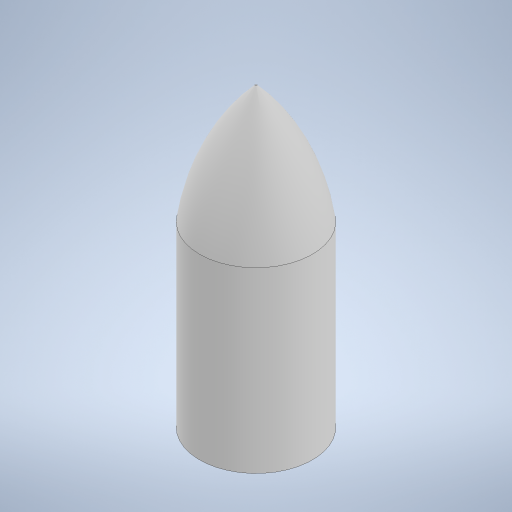
# Autodesk Inventor part: 물로켓탄두1
Saved by Autodesk Inventor 2023 (Build 270158000, 158)
## iProperties
Created: 2023-08-29
Part Number: 물로켓탄두1
Material: 일반
Document SubType Name: Modeling
Designer: rlatk
Density: 1 g/cm^3
Appearance: 기본값
Author: rlatk
Autodesk Inventor part; units mm, degrees
ref_plane "YZ Plane" through (0, 0, 0) normal (1, 0, 0) x (0, 1, 0)
ref_plane "XZ Plane" through (0, 0, 0) normal (0, 1, 0) x (-1, 0, 0)
ref_plane "XY Plane" through (0, 0, 0) normal (0, 0, 1) x (1, 0, 0)
sketch "스케치1" plane through (0, 0, 0) normal (0, 1, 0) x (-1, 0, 0)
  circle A0 centre (0, 0) radius 45.5
  circle A1 centre (0, 0) radius 47.5
  dimension "d0" = 91
  dimension "d1" = 2
  constraints: 2 centre point, 1 coincident
  measures "d0" diameter of A0
  measures "d1" radial gap between concentric circles of A0 A1
extrude "돌출1" add sketch "스케치1" along normal blind 150
sketch "스케치2" plane through (0, 0, 0) normal (1, 0, 0) x (0, 1, 0)
  line L0 (150, 45.5) -> (150, -45.5) projected
  line L1 (0, 45.5) -> (0, -45.5) projected
  line L2 (150, 45.5) -> (0, 45.5) projected
  line L3 (150, -45.5) -> (0, -45.5) projected
  arc A0 (246.756, 0.7428) -> (150, 45.5) centre (126.1059, -133.1163) ccw
  line L4 (150, -47.5) -> (150, 47.5) projected
  arc A1 (249.7064, 0.7347) -> (150, 47.5) centre (126.1059, -133.1163) ccw
  arc A2 (250.028, 0) -> (249.7064, 0.7347) centre (249.028, 0) ccw
  arc A3 (247.0865, 0) -> (246.756, 0.7428) centre (246.0865, 0) ccw
  line L5 (150, 47.5) -> (150, 45.5)
  line L6 (150, -45.5) -> (150, -47.5)
  line L7 (250.028, 0) -> (247.0865, 0)
  line L8 (-51.4681, 0) -> (308.8084, 0) projected
  line L9 (0, 47.5) -> (150, 47.5) projected
  line L10 (0, -47.5) -> (150, -47.5) projected
  line L11 (0, -47.5) -> (0, 47.5) projected
  point P0 (0, 0)
  point P1 (224.5184, 8.564)
  point P2 (257.3404, -6.7411)
  point P3 (225.3563, -10.3608)
  point P4 (224.5184, -8.564)
  point P5 (257.3404, 6.7411)
  dimension "d5" = 1
  constraints: 8 point on circle, 6 end point, 4 centre point, 2 tangent, 2 vertical, 1 equal radius, 3 other
  measures "d5" radius of A2
revolve "회전1" add sketch "스케치2" angle 360 about axis through (0, -10, 0) along (0, 1, 0) contours L4 A1 A2 L7 A3 A0
